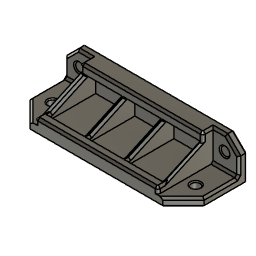
Parametric_Wago_Mount v4 (Autodesk Fusion 360 design; units mm, degrees)
Autodesk Fusion 360 part; units mm, degrees
sketch "MainBody" plane through (0, 0, 0) normal (1, 0, 0) x (0, 1, 0)
  line L0 (0, 0) -> (24.5, 0) construction
  line L1 (24.5, 0) -> (24.5, 15) construction
  line L2 (24.5, 15) -> (0, 15) construction
  line L3 (0, 15) -> (0, 0) construction
  line L4 (0, 15) -> (21.5, 15) construction
  line L5 (21.5, 15) -> (21.5, 3.6) construction
  line L6 (21.5, 3.6) -> (0, 3.6) construction
  line L7 (0, 3.6) -> (0, 15) construction
  line L8 (21.5, 3.6) -> (3, 3.6) construction
  line L9 (3, 3.6) -> (3, 11.85) construction
  line L10 (3, 11.85) -> (21.5, 11.85) construction
  line L11 (21.5, 11.85) -> (21.5, 3.6) construction
  line L12 (3, 3.6) -> (0, 3.6) construction
  line L13 (0, 3.6) -> (0, 5.4) construction
  line L14 (0, 5.4) -> (3, 5.4) construction
  line L15 (3, 5.4) -> (3, 3.6) construction
  line L16 (21.5, 15) -> (17.5, 15) construction
  line L17 (17.5, 15) -> (17.5, 11.85) construction
  line L18 (17.5, 11.85) -> (21.5, 11.85) construction
  line L19 (21.5, 11.85) -> (21.5, 15) construction
  line L20 (24.5, 15) -> (24.5, 0)
  line L21 (24.5, 0) -> (0, 0)
  line L22 (0, 5.4) -> (0, 0)
  line L23 (0, 5.4) -> (3, 5.4)
  line L24 (17.5, 11.85) -> (17.5, 15)
  line L25 (17.5, 15) -> (24.5, 15)
  line L26 (21.5, 3.6) -> (21.5, 11.85)
  line L27 (21.5, 11.85) -> (17.5, 11.85)
  line L28 (21.5, 3.6) -> (3, 3.6)
  line L29 (3, 5.4) -> (3, 3.6)
  line L30 (0, 3.6) -> (24.5, 3.6)
  line L31 (3, 5.4) -> (4.6, 5.4)
  line L32 (4.6, 5.4) -> (17.5, 11.25)
  line L33 (4.6, 5.4) -> (20.9055, 5.4) construction
  line L34 (17.5, 11.85) -> (17.5, 11.25)
  dimension "d10" = 24.5
  dimension "d11" = 15
  dimension "d12" = 21.5
  dimension "d13" = 11.4
  dimension "d14" = 18.5
  dimension "d15" = 8.25
  dimension "d16" = 3
  dimension "d17" = 1.8
  dimension "d18" = 4
  dimension "d53" = 3.15
  dimension "d54" = 1.6
  dimension "d94" = 3.75
  constraint horizontal L0
  constraint vertical L1
  constraint horizontal L2
  constraint vertical L3
  constraint coincident L0.start L3.end
  constraint horizontal L4
  constraint vertical L5
  constraint horizontal L6
  constraint vertical L7
  constraint horizontal L8
  constraint vertical L9
  constraint horizontal L10
  constraint vertical L11
  constraint horizontal L12
  constraint vertical L13
  constraint horizontal L14
  constraint vertical L15
  constraint horizontal L16
  constraint vertical L17
  constraint horizontal L18
  constraint vertical L19
  constraint coincident L20 L30.end
  constraint perpendicular L20 L30
  constraint perpendicular L9 L31
  constraint horizontal L33
  constraint perpendicular L10 L34
  measures "d10" distance of L0.start L0.end
  measures "d11" distance of L0.start L2.end
  measures "d12" distance of L2.end L4.end
  measures "d13" distance of L2.end L6.end
  measures "d14" distance of L5.end L8.end
  measures "d15" distance of L5.end L10.end
  measures "d16" distance of L8.end L6.end
  measures "d17" distance of L8.end L14.end
  measures "d18" distance of L4.end L16.end
  measures "d53" distance of L2 L18
  measures "d54" distance of L14.end L31.end
  measures "d94" distance of L4 L32.end
extrude "Extrude1" add sketch "MainBody" against normal blind 2 makes body 1 in component "MainWagoMount"
extrude "Extrude2" add 1 faces at (0, 15.5333, 5.55) along direction (1, 0, 0) blind 45.6 on bodies 1 bodies 1 in component "MainWagoMount"
extrude "Extrude3" cut sketch "MainBody" along normal blind 13.2 contours L26 L27 L28 L29 L30 L31 L32 L34 bodies 1 in component "MainWagoMount"
chamfer "Chamfer1" distance 0.8 angle 45 6 edges at (13.2, 11.05, 8.325) (13.2, 17.5, 11.55) (0, 17.5, 11.55) (0, 11.05, 8.325) (0, 3.8, 5.4) (13.2, 3.8, 5.4) on bodies 1 in component "MainWagoMount"
pattern_linear "R-Pattern1" count 3 spacing 15.2 along (1, 0, 0) of "Extrude3", "Chamfer1" in component "MainWagoMount"
sketch "MountingTab" plane through (-2, 0, 0) normal (-1, 0, 0) x (0, -1, 0)
  line L0 (-17.5, 11.25) -> (-17.5, 15)
  line L1 (-17.5, 15) -> (-24.5, 15)
  line L2 (-24.5, 15) -> (-24.5, 0)
  line L3 (-24.5, 0) -> (0, 0)
  line L4 (0, 0) -> (0, 5.4)
  line L5 (0, 5.4) -> (-4.6, 5.4)
  line L6 (-4.6, 5.4) -> (-17.5, 11.25)
  line L7 (-24.5, 3) -> (0, 3) construction
  line L8 (-21.5, 15) -> (-21.5, 0) construction
  line L9 (-21.5, 15) -> (-21.5, 3)
  line L10 (0, 3) -> (-21.5, 3)
  dimension "d68" = -3
  dimension "d69" = -3
  constraint coincident L7 L9.end
  constraint coincident L8 L9.end
  constraint perpendicular L7 L9
extrude "Extrude1'" add sketch "MountingTab" along normal blind 10 separate body contours L1 L2 L3 L4 L9 L10 makes body 2 in component "End"
sketch "Sketch1" plane through (0, 0, 3) normal (0, 0, 1) x (-1, 0, 0) in component "End"
  line L0 (2, 0) -> (2, -21.5)
  line L1 (2, -21.5) -> (12, -21.5)
  line L2 (12, -21.5) -> (12, 0)
  line L3 (12, 0) -> (2, 0)
  line L4 (6, 0) -> (6, -21.5) construction
  circle A0 centre (6, -10.75) radius 1.7
  line L5 (2, -10.75) -> (6, -10.75) construction
  circle A1 centre (6, -10.75) radius 5 construction
  dimension "d72" = -4
  dimension "d73" = 3.4
  dimension "d80" = 10
  constraint midpoint L4 A0.centre
  constraint midpoint L0 L5.start
  constraint coincident A0.centre L5.end
  constraint perpendicular L4 L5
  measures "d73" diameter of A0
  measures "d80" diameter of A1
sketch "Sketch2" plane through (0, 21.5, 0) normal (0, -1, 0) x (1, 0, 0) in component "End"
  line L0 (-2, 3) -> (-2, 15)
  line L1 (-2, 15) -> (-12, 15)
  line L2 (-12, 15) -> (-12, 3)
  line L3 (-12, 3) -> (-2, 3)
  line L4 (-6, 3) -> (-7, 15) construction
  circle A0 centre (-6.5, 9) radius 1.7
  circle A1 centre (-6.5, 9) radius 3 construction
  point P0 (-6, 3)
  dimension "d74" = 3.4
  dimension "d79" = 6
  constraint coincident P0 L4.start
  constraint midpoint L1 L4.end
  constraint midpoint L4 A0.centre
  constraint concentric A0 A1
  measures "d74" diameter of A0
  measures "d79" diameter of A1
extrude "Extrude2'" cut sketch "Sketch2" against normal blind 0.4 contours A0 bodies 2 in component "End"
extrude "Extrude3'" cut sketch "Sketch1" against normal blind 5 contours A0 bodies 2 in component "End"
chamfer "Chamfer1'" distance 8 angle 45 1 edges at (-12, 0, 1.5) on bodies 2 in component "End"
chamfer "Chamfer2" distance 5 angle 45 1 edges at (-12, 23, 15) on bodies 2 in component "End"
chamfer "Chamfer3" distance 0.4 angle 45 2 edges at (-8.085, 21.5, 9.6147) (-4.415, 10.1353, 3) on bodies 2 in component "End"
chamfer "Chamfer5" distance 0.8 angle 45 1 edges at (-7, 21.5, 3) on bodies 2 in component "End"
ref_plane "WorkPlane2" through (21.8, 12.25, 7.5) normal (-1, 0, 0) x (0, 0, 1)
chamfer "Chamfer6" distance 0.8 angle 45 6 edges at (-8, 4, 3) (-12, 14.35, 3) (-12, 21.1, 3.4) (-12, 21.5, 6.9) (-9.5, 21.5, 12.5) (-4.5, 21.5, 15) on bodies 2 in component "End"
mirror "MirrorComponent3" about plane through (0, 0, 0) normal (0, 0, 1) of bodies 2 makes body 3 in component "End(Mirror)"
combine "Combine2" operation add target body 1 tool bodies 2 3 body 3 seen with x (-1, 0, 0) y (0, 1, 0) z (0, 0, -1) at (43.6, 0, 0) in component "MainWagoMount"
fillet "Fillet1" radius 1 4 edges at (45.6, 0, 4.2) (-2, 0, 4.2) (45.6, 17.5, 13.125) (-2, 17.5, 13.125) on bodies 1 in component "MainWagoMount"
chamfer "Chamfer4" distance 0.8 angle 45 10 edges at (21.8, 0, 5.4) (45.3071, 0.2929, 5.4) (45.6, 2.8, 5.4) (-2, 2.8, 5.4) (-1.7071, 0.2929, 5.4) (-1.7071, 17.7929, 15) (-2, 20.4, 15) (45.6, 20.4, 15) (45.3071, 17.7929, 15) (21.8, 17.5, 15) on bodies 1 in component "MainWagoMount"
chamfer "Chamfer3'" distance 0.4 angle 45 2 faces at (12.2, 24.5, 5) (30.6513, 20.3021, 0) on bodies 1 in component "MainWagoMount"
component "MainWagoMount" placed x (1, 0, 0) y (0, 1, 0) z (0, 0, 1) at (0, 0, 0)
equation "WagoSize = 2"
equation "WagoExtrude = ( ( 5.5 * WagoSize ) * 1 mm ) + 2.2 mm"
equation "NumOfWagos = 3"
equation "PatternSpacing = WagoExtrude + 2 mm"
equation "MidPlane = ( ( PatternSpacing * NumOfWagos ) / 2 ) + 1 mm"
equation "FullExtrude = PatternSpacing * NumOfWagos"
equation "ExtrusionSize = 15 mm"
equation "MountingScrew = 5 mm"
equation "TopOrSide = 1" comment "0 if mounted to the side (in extrusion) 1 if Mounted on top on a flat panel"
equation "SideExtrusion = ( if(TopOrSide < 1; 5; 0.4) ) * 1 mm"
equation "BottomExtrusion = ( if(TopOrSide > 0; 5; 0.4) ) * 1 mm"
equation "ScrewCheck = ( ( if(ExtrusionSize < 20 mm; if(MountingScrew > 3 mm; 3 mm; MountingScrew); MountingScrew) ) )"
equation "d59 = PatternSpacing * NumOfWagos"
equation "d61 = WagoExtrude"
equation "d64 = NumOfWagos"
equation "d66 = PatternSpacing"
equation "d70 = ExtrusionSize - 5 mm"
equation "d72 = ( -ExtrusionSize + 7 mm ) / 2"
equation "d73 = ScrewCheck + 0.4 mm"
equation "d74 = ScrewCheck + 0.4 mm"
equation "d75 = -SideExtrusion"
equation "d77 = -BottomExtrusion"
equation "d79 = ScrewCheck * 2"
equation "d86 = -MidPlane"
equation "WagoSizeExtrudeValue = 1 mm"
